# Autodesk Inventor part: 同步皮带
Saved by Autodesk Inventor 2015 (Build 190159000, 159)
## iProperties
Created: 2017-05-28
Part Number: 同步皮带
Material: Rubber
Document SubType Name: Modeling
Designer: Administrator
Density: 1 g/cm^3
Appearance: Rubber - Black - Version 1.1
CustomPartVersion: 1
Author: Administrator
Autodesk Inventor part; units mm, degrees
sketch "草图路径" plane through (0, 0, 0) normal (0, 0, 1) x (1, 0, 0)
  arc A0 (-29.2363, 8.0302) -> (28.5834, -10.111) centre (0, 0) ccw
  arc A1 (115.6836, 308.3782) -> (56.271, 319.3456) centre (85.5072, 311.3155) ccw
  arc A2 (105.1569, 206.3581) -> (106.2189, 211.1407) centre (86.1013, 213.0988) ccw
  line L0 (105.1569, 206.3581) -> (28.5834, -10.111)
  line L1 (-29.2363, 8.0302) -> (56.271, 319.3456)
  line L2 (115.6836, 308.3782) -> (106.2189, 211.1407)
  constraints: 6 end point, 6 point on circle, 3 centre point
ref_plane "截面平面" through (28.5834, -10.111, 0) normal (0.3335, 0.9428, 0) x (0, 0, 1)
ref_plane "工作平面2" through (0, 0, 0) normal (-1, 0, 0) x (0, 0, 1)
ref_plane "工作平面3" through (85.5072, 311.3155, 0) normal (-0.5284, -0.849, 0) x (0, 0, 1)
ref_plane "工作平面4" through (86.1013, 213.0988, 0) normal (0.6175, 0.7866, 0) x (0, 0, 1)
sketch "截面" plane through (28.5834, -10.111, 0) normal (0.3335, 0.9428, 0) x (0, 0, 1)
  line L0 (-9.525, 1.3462) -> (9.525, 1.3462)
  line L1 (9.525, 1.3462) -> (9.525, -0.6858)
  line L2 (9.525, -0.6858) -> (-9.525, -0.6858)
  line L3 (-9.525, -0.6858) -> (-9.525, 1.3462)
  line L4 (-9.525, 0) -> (9.525, 0) construction
  point P0 (0, 0)
  point P1 (0, 0)
  dimension "d0" = 19.05
  dimension "d4" = 0.6858
  dimension "d5" = 1.3462
  constraints: 10 end point, 2 parallel, 2 point on line, 1 coincident, 1 horizontal, 1 midpoint, 1 perpendicular, 1 other
  measures "d0" distance between parallel lines of L1 L3
  measures "d4" distance between parallel lines of L2 L4
  measures "d5" distance between parallel lines of L4 L0
sweep "皮带" add profiles "截面" path "草图路径"
equation "\"d0\" = da_B"
equation "\"d4\" = da_a"
equation "\"d5\" = da_a2"
equation "\"da_B\" = 19.05"
equation "\"da_pb\" = 12.7"
equation "\"da_L\" = 838.2"
equation "\"da_a\" = 0.6858"
equation "\"da_S\" = 6.1214"
equation "\"da_Beta\" = 20deg"
equation "\"da_Ht\" = 2.286"
equation "\"da_H\" = 4.318"
equation "\"da_a2\" = 1.3462"
body "Solid1"
